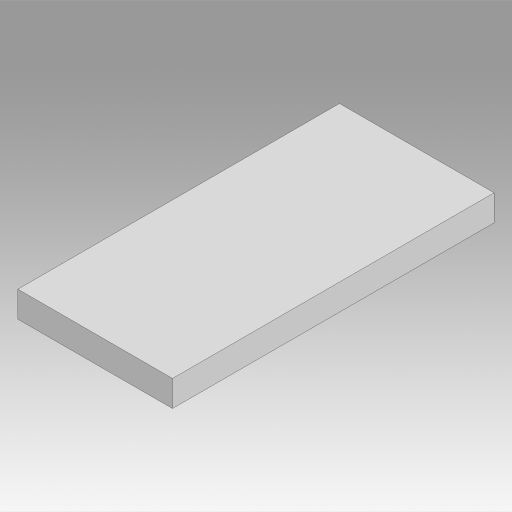
# Autodesk Inventor part: lid
Saved by Autodesk Inventor 2023 (Build 270158000, 158)
## iProperties
Created: 2025-08-22
Part Number: lid
Material: Generic
Document SubType Name: Modeling
Designer: NELLY NDUNG'U
Density: 1 g/cm^3
Appearance: Default
Author: NELLY NDUNG'U
Autodesk Inventor part; units mm, degrees
ref_plane "YZ Plane" through (0, 0, 0) normal (1, 0, 0) x (0, 1, 0)
ref_plane "XZ Plane" through (0, 0, 0) normal (0, 1, 0) x (-1, 0, 0)
ref_plane "XY Plane" through (0, 0, 0) normal (0, 0, 1) x (1, 0, 0)
sketch "Sketch1" plane through (0, 0, 0) normal (0, 1, 0) x (-1, 0, 0)
  line L0 (7.5405, 15.6819) -> (-7.5405, 15.6819)
  line L1 (-7.5405, 15.6819) -> (-7.5405, -15.6819)
  line L2 (-7.5405, -15.6819) -> (7.5405, -15.6819)
  line L3 (7.5405, -15.6819) -> (7.5405, 15.6819)
  line L4 (7.5405, 15.6819) -> (-7.5405, -15.6819) construction
  line L5 (-7.5405, 15.6819) -> (7.5405, -15.6819) construction
  point P0 (0, 0)
  constraints: 12 end point, 2 midpoint, 2 parallel, 1 horizontal, 1 perpendicular
extrude "Extrusion1" add sketch "Sketch1" along normal blind 2.54
body "Solid1"
